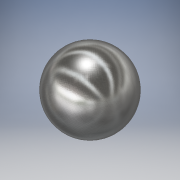
# Autodesk Inventor part: ballbearing
Saved by Autodesk Inventor 2019 (Build 230136000, 136)
## iProperties
Created: 2020-12-18
Part Number: ballbearing
Material: Generic
Document SubType Name: Modeling
Designer: saeva
Density: 1 g/cm^3
Appearance: Default
Author: saeva
Autodesk Inventor part; units mm, degrees
ref_plane "YZ Plane" through (0, 0, 0) normal (1, 0, 0) x (0, 1, 0)
ref_plane "XZ Plane" through (0, 0, 0) normal (0, 1, 0) x (-1, 0, 0)
ref_plane "XY Plane" through (0, 0, 0) normal (0, 0, 1) x (1, 0, 0)
sketch "Sketch1" plane through (0, 0, 0) normal (1, 0, 0) x (0, 1, 0)
  line L0 (0, 0) -> (28.8377, 0)
  arc A0 (28.8377, 0) -> (0, 0) centre (14.4188, 0) ccw
  dimension "d1" = 90
  constraints: 2 end point, 2 point on circle, 1 centre point, 1 horizontal, 1 midpoint
revolve "Revolution1" add sketch "Sketch1" angle 360 about axis through (0, 0, 0) along (0, 1, 0)
body "Solid1"
